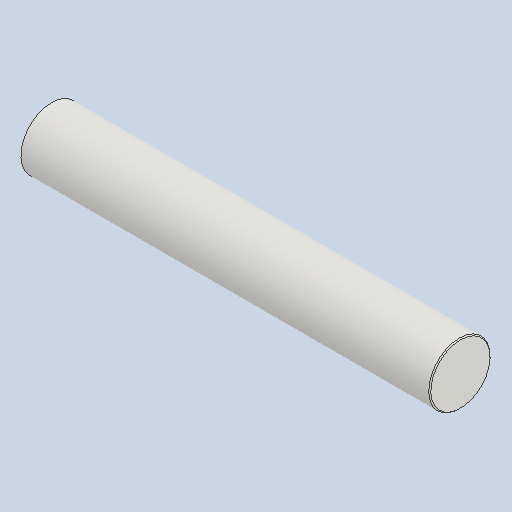
# Autodesk Inventor part: Shaft
Saved by Autodesk Inventor 2022 (Build 260153000, 153)
## iProperties
Created: 2022-02-01
Part Number: Shaft
Material: Steel
Document SubType Name: Modeling
Designer: br4ch
Density: 1 g/cm^3
Appearance: Steel
CustomPartVersion: 1
Author: br4ch
Length: 40,000 mm
Autodesk Inventor part; units mm, degrees
ref_plane "Start Plane" through (0, 0, 0) normal (1, 0, 0) x (0, 1, 0)
ref_plane "XZ Plane" through (0, 0, 0) normal (0, 1, 0) x (-1, 0, 0)
ref_plane "XY Plane" through (0, 0, 0) normal (0, 0, 1) x (1, 0, 0)
sketch "Main Sketch" plane through (0, 0, 0) normal (0, 0, 1) x (1, 0, 0)
  line L0 (0, 0) -> (40, 0)
  line L1 (0, 0) -> (0, 3)
  line L2 (0, 3) -> (40, 3)
  line L3 (40, 3) -> (40, 0)
  dimension "d3" = 6
  constraints: 8 end point, 2 horizontal, 2 vertical
  measures "d3" diameter of L2 L0
revolve "Revolution1" add sketch "Main Sketch" angle 360 about axis through (0, 0, 0) along (1, 0, 0)
chamfer "Chamfer1" distance 0.1 angle 45 1 edges at (40, -3, 0) measured on face at (13.3333, 2.9612, -0.4812)
equation "\"Length\" = 40"
body "Solid1"
